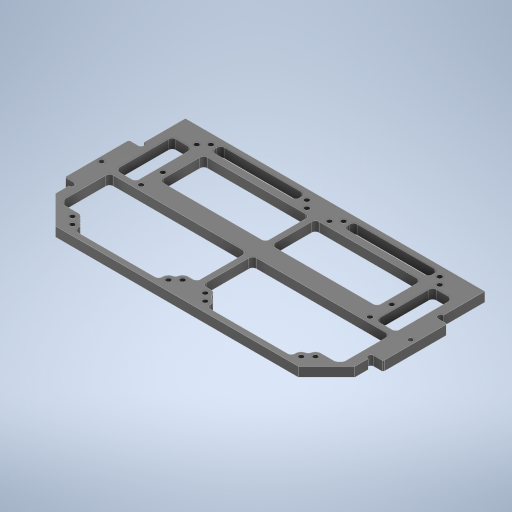
# Autodesk Inventor part: TorsoElectronicBoxBoardMountFrame
Saved by Autodesk Inventor 2024.2 (Build 282272000, 272)
## iProperties
Created: 2024-01-11
Part Number: TorsoElectronicBoxBoardMountFrame
Material: Acetal Resin, Black
Document SubType Name: Modeling
Designer: Masato Kubotera
Density: 1.425 g/cm^3
Appearance: Smooth - Black
Vendor: meviy
Mass: 32.4012 g
Surface Area: 177.402 cm^2
Volume: 22.7377 cm^3
Author: Masato Kubotera
Autodesk Inventor part; units mm, degrees
ref_plane "YZ Plane" through (0, 0, 0) normal (1, 0, 0) x (0, 1, 0)
ref_plane "XZ Plane" through (0, 0, 0) normal (0, 1, 0) x (-1, 0, 0)
sketch "Sketch1" plane through (0, 0, 0) normal (0, 0, 1) x (1, 0, 0)
  line L0 (-42, -79.5) -> (42, -79.5)
  line L1 (42, -79.5) -> (42, 79.5)
  line L2 (42, 79.5) -> (-42, 79.5) construction
  line L3 (-42, 79.5) -> (-42, -79.5)
  line L4 (-42, -79.5) -> (42, 79.5) construction
  line L5 (42, -79.5) -> (-42, 79.5) construction
  line L6 (-42, 0) -> (42, 0)
  line L7 (-17, 84.5) -> (17, 84.5)
  line L8 (17, 84.5) -> (17, 79.5)
  line L9 (-17, 84.5) -> (-17, 79.5)
  arc A0 (-20, 79.5) -> (-17, 79.5) centre (-18.5, 79.5) ccw
  line L10 (17, 84.5) -> (17, 79.5)
  arc A1 (17, 79.5) -> (20, 79.5) centre (18.5, 79.5) ccw
  line L11 (0, 79.5) -> (0, 84.5) construction
  line L12 (0, -79.5) -> (0, 70) construction
  line L13 (-33, 6) -> (33, 6) construction
  line L14 (33, 6) -> (33, 64.5) construction
  line L15 (33, 64.5) -> (-33, 64.5) construction
  line L16 (-33, 64.5) -> (-33, 6) construction
  line L17 (-33, 6) -> (33, 64.5) construction
  line L18 (33, 6) -> (-33, 64.5) construction
  line L19 (-41, 1.75) -> (41, 1.75) construction
  line L20 (41, 1.75) -> (41, 68.75) construction
  line L21 (41, 68.75) -> (-41, 68.75) construction
  line L22 (-41, 68.75) -> (-41, 1.75) construction
  line L23 (-41, 1.75) -> (41, 68.75) construction
  line L24 (41, 1.75) -> (-41, 68.75) construction
  line L25 (-41, 35.25) -> (41, 35.25) construction
  line L26 (5.25, 74.5) -> (26.9289, 74.5)
  arc A2 (36.9, 12.7462) -> (39, 14.7437) centre (37, 14.7437) ccw
  arc A3 (28, 1.5) -> (30, 3.5) centre (28, 3.5) ccw
  line L27 (-42, 79.5) -> (-20, 79.5)
  line L28 (20, 79.5) -> (42, 79.5)
  line L29 (-31, 0) -> (0, 0) construction
  circle A4 centre (-33, 6) radius 3 construction
  line L30 (5.25, 1.5) -> (28, 1.5)
  arc A5 (5.25, 74.5) -> (3.25, 72.5) centre (5.25, 72.5) ccw
  line L31 (-28, 1.5) -> (-8.5, 1.5)
  line L32 (-6.5, 3.5) -> (-6.5, 55.75)
  line L33 (-8.5, 57.75) -> (-28, 57.75)
  line L34 (-30, 55.75) -> (-30, 3.5)
  arc A6 (-30, 3.5) -> (-28, 1.5) centre (-28, 3.5) ccw
  arc A7 (-8.5, 1.5) -> (-6.5, 3.5) centre (-8.5, 3.5) ccw
  arc A8 (-6.5, 55.75) -> (-8.5, 57.75) centre (-8.5, 55.75) ccw
  arc A9 (-28, 57.75) -> (-30, 55.75) centre (-28, 55.75) ccw
  arc A10 (33.8266, 60.0766) -> (36.9, 57.7538) centre (36.75, 60.75) ccw
  arc A11 (39, 55.7563) -> (36.9, 57.7538) centre (37, 55.7563) ccw
  line L35 (39, 55.7563) -> (39, 14.7437)
  arc A12 (36.9, 12.7462) -> (33.8266, 10.4234) centre (36.75, 9.75) ccw
  arc A13 (3.25, 3.5) -> (5.25, 1.5) centre (5.25, 3.5) ccw
  line L36 (-28, 63.75) -> (-1.75, 63.75)
  line L37 (0.25, 65.75) -> (0.25, 72.5)
  line L38 (-1.75, 74.5) -> (-28, 74.5)
  line L39 (-30, 72.5) -> (-30, 65.75)
  line L40 (-37, 12.75) -> (-35.75, 12.75)
  line L41 (-33.75, 14.75) -> (-33.75, 55.75)
  line L42 (-35.75, 57.75) -> (-37, 57.75)
  line L43 (-39, 55.75) -> (-39, 14.75)
  circle A14 centre (-36.75, 9.75) radius 3 construction
  circle A15 centre (-36.75, 60.75) radius 3 construction
  arc A16 (-30, 65.75) -> (-28, 63.75) centre (-28, 65.75) ccw
  arc A17 (-1.75, 63.75) -> (0.25, 65.75) centre (-1.75, 65.75) ccw
  arc A18 (0.25, 72.5) -> (-1.75, 74.5) centre (-1.75, 72.5) ccw
  arc A19 (-28, 74.5) -> (-30, 72.5) centre (-28, 72.5) ccw
  arc A20 (-33.75, 55.75) -> (-35.75, 57.75) centre (-35.75, 55.75) ccw
  arc A21 (-37, 57.75) -> (-39, 55.75) centre (-37, 55.75) ccw
  arc A22 (-39, 14.75) -> (-37, 12.75) centre (-37, 14.75) ccw
  arc A23 (-35.75, 12.75) -> (-33.75, 14.75) centre (-35.75, 14.75) ccw
  line L44 (27, 79.5) -> (42, 64.5)
  line L45 (29.4142, 72.8431) -> (28.3431, 73.9142)
  arc A24 (30, 71.4289) -> (29.4142, 72.8431) centre (28, 71.4289) ccw
  arc A25 (28.3431, 73.9142) -> (26.9289, 74.5) centre (26.9289, 72.5) ccw
  circle A26 centre (33, 6) radius 3 construction
  line L46 (0.25, 9.75) -> (36.75, 9.75) construction
  line L47 (36.75, 9.75) -> (36.75, 60.75) construction
  line L48 (36.75, 60.75) -> (0.25, 60.75) construction
  line L49 (0.25, 60.75) -> (0.25, 9.75) construction
  line L50 (0.25, 9.75) -> (36.75, 60.75) construction
  line L51 (36.75, 9.75) -> (0.25, 60.75) construction
  arc A27 (32.3266, 8.9234) -> (30, 6) centre (33, 6) ccw
  line L52 (30, 3.5) -> (30, 6)
  arc A28 (33.8828, 61.6328) -> (36.9, 57.7538) centre (36.75, 60.75) ccw
  arc A29 (30, 64.5) -> (32.3266, 61.5766) centre (33, 64.5) ccw
  line L53 (30, 71.4289) -> (30, 64.5)
  line L54 (3.25, 3.5) -> (3.25, 72.5)
  circle A30 centre (0.25, 60.75) radius 3 construction
  arc A31 (33.8266, 60.0766) -> (32.3266, 61.5766) centre (31.8776, 59.6276) ccw
  arc A32 (32.3266, 8.9234) -> (33.8266, 10.4234) centre (31.8776, 10.8724) ccw
  line L55 (-33.75, -53.5) -> (-2.75, -53.5) construction
  line L56 (-2.75, -53.5) -> (-2.75, 53.5) construction
  line L57 (-2.75, 53.5) -> (-33.75, 53.5) construction
  line L58 (-33.75, 53.5) -> (-33.75, -53.5) construction
  line L59 (-33.75, -53.5) -> (-2.75, 53.5) construction
  line L60 (-2.75, -53.5) -> (-33.75, 53.5) construction
  line L61 (-18.25, -53.5) -> (-18.25, 53.5) construction
  point P0 (0, 0)
  point P1 (0, 35.25)
  point P2 (0, 82)
  point P3 (0.1, 0)
  point P4 (-30, 63.75)
  point P5 (0.25, 74.5)
  point P6 (0.25, 63.75)
  point P7 (-30, 74.5)
  point P8 (-39, 12.75)
  point P9 (-33.75, 57.75)
  point P10 (-33.75, 12.75)
  point P11 (-39, 57.75)
  point P12 (18.5, 35.25)
  point P13 (-11.25, 60.75)
  point P14 (-18.25, 0)
  dimension "d1" = 159
  dimension "d2" = 1.5
  dimension "d3" = 5
  dimension "d36" = 25
  dimension "d42" = 58.5
  dimension "d43" = 66
  dimension "d44" = 82
  dimension "d45" = 67
  dimension "d67" = 5
  dimension "d70" = 42
  dimension "d71" = 84
  dimension "d73" = 25
  dimension "d75" = 12
  dimension "d102" = 6
  dimension "d108" = 3
  dimension "d116" = 3
  dimension "d118" = 6
  dimension "d122" = 2
  dimension "d147" = 15
  dimension "d148" = 45
  dimension "d150" = 3
  dimension "d151" = 51
  dimension "d153" = 36.5
  dimension "d156" = 25.5
  dimension "d159" = 11.5
  dimension "d160" = 19.5
  dimension "d161" = 31
  dimension "d162" = 107
  dimension "d163" = 3
  constraints: 124 end point, 58 point on circle, 46 tangent, 33 centre point, 27 point on line, 25 equal radius, 20 midpoint, 17 parallel, 12 coincident, 11 horizontal, 9 symmetric about line, 8 collinear, 8 perpendicular, 6 vertical, 8 other
  measures "d1" distance of L1.end L0.end
  measures "d2" radius of A0
  measures "d3" distance of L7.start L9.end
  measures "d36" distance between parallel lines of L8 L1
  measures "d42" distance of L15.end L13.start
  measures "d43" distance of L14.end L15.end
  measures "d44" distance of L21.end L20.end
  measures "d45" distance of L19.end L20.end
  measures "d67" distance between parallel lines of L2 L26
  measures "d70" distance between parallel lines of L1 L12
  measures "d71" distance between parallel lines of L1 L3
  measures "d73" distance between parallel lines of L9 L3
  measures "d75" diameter of point (-33, 6) L6
  measures "d102" diameter of A4
  measures "d108" diameter of L30 L6
  measures "d116" distance between parallel lines of L1 L35
  measures "d118" diameter of A12
  measures "d122" radius of A3
  measures "d147" distance of L1.end L44.end
  measures "d148" angle of L1 L44
  measures "d150" distance between parallel lines of L44 L45
  measures "d151" distance of A10.centre point (36.75, 9.75)
  measures "d153" distance of L47.end L48.end
  measures "d156" distance of point (-11.25, 60.75) A15.centre
  measures "d159" distance of point (0.25, 60.75) point (-11.25, 60.75)
  measures "d160" diameter of point (36.75, 9.75) L6
  measures "d161" distance of L57.end L56.end
  measures "d162" distance of L56.end L55.end
  measures "d163" distance between parallel lines of L37 L54
extrude "Extrusion1" add sketch "Sketch1" against normal blind 5 contours L3 L27 A0 L9 L7 L8 A1 L28 L44 L1 L6
chamfer "C0.5" distance 0.5 angle 45 2 edges at (17, 84.5, -2.5) (-17, 84.5, -2.5)
hole "M3" at (-33, 6, 0) at (-33, 64.5, 0) at (33, 6, 0) at (33, 64.5, 0) at (36.75, 9.75, 0) at (36.75, 60.75, 0) at (-36.75, 9.75, 0) at (-36.75, 60.75, 0) at (0.25, 60.75, 0) at (-11.25, 60.75, 0) direction (0, 0, -1) diameter 2.459 end through all thread size "M3x0.5" class "6H" standard "ANSI Metric M Profile"
hole "Phi2.5" at (0, 82, 0) direction (0, 0, -1) diameter 2.5 end through all
mirror "Mirror1" about plane through (0, 0, 0) normal (0, 1, 0)
ref_plane "Work Plane1" through (-18.25, 3.5, 0) normal (1, 0, 0) x (0, 0, -1)
body "Solid1"
